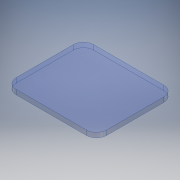
# Autodesk Inventor part: PayloadGermination_Sponge
Saved by Autodesk Inventor 2018 (Build 220112000, 112)
## iProperties
Created: 2018-07-29
Part Number: PayloadGermination_Sponge
Material: Water
Document SubType Name: Modeling
Designer: Bradley
Density: 0.9983 g/cm^3
Appearance: Tropical Blue
Author: Bradley
Autodesk Inventor part; units mm, degrees
ref_plane "YZ Plane" through (0, 0, 0) normal (1, 0, 0) x (0, 1, 0)
ref_plane "XZ Plane" through (0, 0, 0) normal (0, 1, 0) x (-1, 0, 0)
ref_plane "XY Plane" through (0, 0, 0) normal (0, 0, 1) x (1, 0, 0)
sketch "Sketch1" plane through (0, 0, 0) normal (0, 0, 1) x (1, 0, 0)
  line L0 (-29.5, -32.5) -> (29.5, -32.5)
  line L1 (38, -24) -> (38, 24)
  line L2 (29.5, 32.5) -> (-29.5, 32.5)
  line L3 (-38, 24) -> (-38, -24)
  line L4 (-38, -32.5) -> (38, 32.5) construction
  line L5 (38, -32.5) -> (-38, 32.5) construction
  arc A0 (-29.5, 32.5) -> (-38, 24) centre (-29.5, 24) ccw
  arc A1 (-38, -24) -> (-29.5, -32.5) centre (-29.5, -24) ccw
  arc A2 (29.5, -32.5) -> (38, -24) centre (29.5, -24) ccw
  arc A3 (38, 24) -> (29.5, 32.5) centre (29.5, 24) ccw
  point P0 (0, 0)
  dimension "d0" = 76
  dimension "d1" = 65
  dimension "d2" = 8.5
  constraints: 12 end point, 8 point on circle, 8 point on line, 8 tangent, 4 centre point, 3 equal radius, 2 midpoint, 2 parallel, 1 horizontal, 1 perpendicular
  measures "d0" distance of L5.end L4.end
  measures "d1" distance of L4.end L5.start
  measures "d2" radius of A0
extrude "Extrusion1" add sketch "Sketch1" along normal mid plane 4
body "Solid1"
